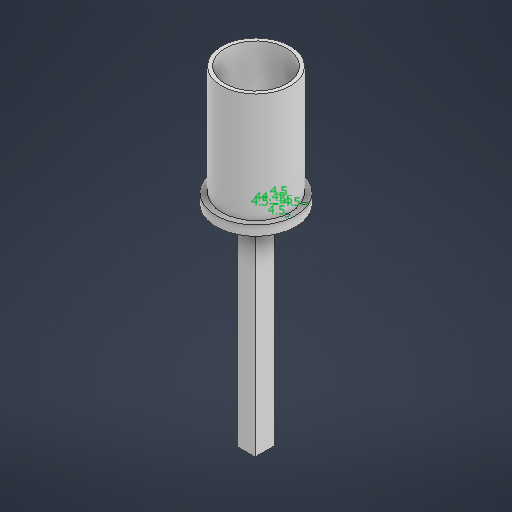
# Autodesk Inventor part: Plunger
Saved by Autodesk Inventor 2025 (Build 290162000, 162)
## iProperties
Created: 2024-06-28
Part Number: Plunger
Material: Generic
Document SubType Name: Modeling
Designer: mayhe
Density: 1 g/cm^3
Appearance: Default
Author: mayhe
Autodesk Inventor part; units mm, degrees
ref_plane "YZ Plane" through (0, 0, 0) normal (1, 0, 0) x (0, 1, 0)
ref_plane "XZ Plane" through (0, 0, 0) normal (0, 1, 0) x (-1, 0, 0)
ref_plane "XY Plane" through (0, 0, 0) normal (0, 0, 1) x (1, 0, 0)
sketch "Sketch1" plane through (0, 0, 0) normal (0, 1, 0) x (-1, 0, 0)
  circle A0 centre (0, 0) radius 110
  circle A1 centre (0, 0) radius 95
  dimension "d0" = 220
  dimension "d1" = 190
  constraints: 2 centre point, 2 coincident
  measures "d0" diameter of A0
  measures "d1" diameter of A1
extrude "Extrusion1" add sketch "Sketch1" along normal blind 330 contours A1
extrude "Extrusion2" add sketch "Sketch1" along normal blind 27
sketch "Sketch2" plane through (0, 330, 0) normal (0, 1, 0) x (1, 0, 0)
  circle A0 centre (0, 0) radius 85
  dimension "d6" = 170
  constraints: 1 centre point, 1 coincident
  measures "d6" diameter of A0
extrude "Extrusion3" cut sketch "Sketch2" against normal blind 300
sketch "Sketch3" plane through (0, 0, 0) normal (0, -1, 0) x (1, 0, 0)
  arc A0 (-25.4, -40.4884) -> (25.4, -40.4884) centre (0, -66) ccw
  circle A1 centre (0, 0) radius 110 projected
  line L0 (25.4, -40.4884) -> (-25.4, -40.4884)
  line L1 (25, -27.5) -> (-25, -27.5)
  line L2 (-25, -27.5) -> (-25, 27.5)
  line L3 (-25, 27.5) -> (25, 27.5)
  line L4 (25, 27.5) -> (25, -27.5)
  line L5 (25, -27.5) -> (-25, 27.5) construction
  line L6 (-25, -27.5) -> (25, 27.5) construction
  arc A2 (41.7582, -27.5) -> (-41.7582, -27.5) centre (0, 0) ccw
  line L7 (25, -27.5) -> (41.7582, -27.5)
  line L8 (-25, -27.5) -> (-41.7582, -27.5)
  dimension "d9" = 72
  dimension "d10" = 66
  dimension "d11" = 50
  dimension "d12" = 55
  dimension "d13" = 100
  constraints: 18 end point, 4 horizontal, 4 point on circle, 2 centre point, 2 midpoint, 2 parallel, 1 coincident, 1 perpendicular
  measures "d9" diameter of A0
  measures "d10" distance of A1.centre A0.centre
  measures "d11" distance of L2.end L3.end
  measures "d12" distance of L1.end L2.end
  measures "d13" diameter of A2
extrude "Extrusion4" add sketch "Sketch3" along normal blind 25 contours L1 L2 L3 L4 | L4 L3 L2 L8 A2 L7
extrude "Extrusion5" add sketch "Sketch3" along normal blind 580 contours L1 L2 L3 L4
extrude "Extrusion6" add sketch "Sketch3" along normal blind 30 contours L0 A0
sketch "Sketch4" plane through (0, -580, 0) normal (0, -1, 0) x (1, 0, 0)
  line L0 (-25, 27.5) -> (25, 27.5) projected
  line L1 (-25, -27.5) -> (25, -27.5)
  line L2 (25, -27.5) -> (25, 27.5)
  line L3 (25, 27.5) -> (-25, 27.5)
  line L4 (-25, 27.5) -> (-25, -27.5)
  line L5 (-25, -27.5) -> (25, 27.5) construction
  line L6 (25, -27.5) -> (-25, 27.5) construction
  line L7 (23, 25.5) -> (23, -25.5)
  line L8 (23, -25.5) -> (-23, -25.5)
  line L9 (-23, -25.5) -> (-23, 25.5)
  line L10 (-23, 25.5) -> (23, 25.5)
  point P0 (0, 0)
  dimension "d20" = 2
  constraints: 20 end point, 4 parallel, 2 midpoint, 2 perpendicular, 1 horizontal, 3 other
  measures "d20" distance between parallel lines of L2 L7
extrude "Extrusion7" cut sketch "Sketch4" against normal through all contours L7 L8 L9 L10
sketch "Sketch5" plane through (0, -30, 0) normal (0, -1, 0) x (1, 0, 0)
  arc A0 (-25.4, -40.4884) -> (25.4, -40.4884) centre (0, -66) ccw projected
  circle A1 centre (0, -66) radius 36
  line L0 (-25.4, -40.4884) -> (25.4, -40.4884) projected
  line L1 (25.4, -40.4884) -> (-25.4, -40.4884)
  circle A2 centre (0, -66) radius 32.5
  line L2 (22.225, -43.775) -> (-22.225, -43.775)
  line L3 (-22.225, -43.775) -> (-22.225, -88.225)
  line L4 (-22.225, -88.225) -> (22.225, -88.225)
  line L5 (22.225, -88.225) -> (22.225, -43.775)
  line L6 (22.225, -43.775) -> (-22.225, -88.225) construction
  line L7 (-22.225, -43.775) -> (22.225, -88.225) construction
  circle A3 centre (-22.225, -88.225) radius 2.25
  circle A4 centre (-22.225, -43.775) radius 2.25
  circle A5 centre (22.225, -88.225) radius 2.25
  circle A6 centre (22.225, -43.775) radius 2.25
  point P0 (0, 0)
  dimension "d23" = 65
  dimension "d24" = 44.45
  dimension "d25" = 4.5
  dimension "d26" = 4.5
  dimension "d27" = 4.5
  dimension "d28" = 4.5
  constraints: 14 end point, 6 centre point, 6 coincident, 3 equal length, 2 midpoint, 1 horizontal, 1 perpendicular
  measures "d23" diameter of A2
  measures "d24" distance of L3.end L2.end
  measures "d25" diameter of A3
  measures "d26" diameter of A4
  measures "d27" diameter of A5
  measures "d28" diameter of A6
body "Solid1"
